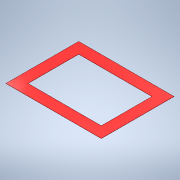
# Autodesk Inventor part: smt_keepout
Saved by Autodesk Inventor 2022 (Build 260153000, 153)
## iProperties
Created: 2022-02-26
Part Number: smt_keepout
Material: Generic
Document SubType Name: Modeling
Designer: Caleb
Density: 1 g/cm^3
Appearance: Light Red
Author: Caleb
Autodesk Inventor part; units mm, degrees
ref_plane "YZ Plane" through (0, 0, 0) normal (1, 0, 0) x (0, 1, 0)
ref_plane "XZ Plane" through (0, 0, 0) normal (0, 1, 0) x (-1, 0, 0)
ref_plane "XY Plane" through (0, 0, 0) normal (0, 0, 1) x (1, 0, 0)
sketch "Sketch1" plane through (0, 0, 0) normal (0, 1, 0) x (-1, 0, 0)
  line L0 (-28.25, -21.55) -> (28.25, -21.55)
  line L1 (28.25, -21.55) -> (28.25, 21.55)
  line L2 (28.25, 21.55) -> (-28.25, 21.55)
  line L3 (-28.25, 21.55) -> (-28.25, -21.55)
  line L4 (-28.25, -21.55) -> (28.25, 21.55) construction
  line L5 (28.25, -21.55) -> (-28.25, 21.55) construction
  point P0 (0, 0)
  dimension "d0" = 43.1
  dimension "d1" = 56.5
  constraints: 12 end point, 2 midpoint, 2 parallel, 1 horizontal, 1 perpendicular
  measures "d0" distance of L0.end L1.end
  measures "d1" distance of L1.end L2.end
extrude "Extrusion1" add sketch "Sketch1" along normal blind 0.1
sketch "Sketch2" plane through (0, 0.1, 0) normal (0, 1, 0) x (1, 0, 0)
  line L0 (21.75, 15.05) -> (-21.75, 15.05)
  line L1 (-21.75, 15.05) -> (-21.75, -15.05)
  line L2 (-21.75, -15.05) -> (21.75, -15.05)
  line L3 (21.75, -15.05) -> (21.75, 15.05)
  line L4 (21.75, 15.05) -> (-21.75, -15.05) construction
  line L5 (-21.75, 15.05) -> (21.75, -15.05) construction
  line L6 (-28.25, -21.55) -> (28.25, -21.55) projected
  line L7 (-28.25, 21.55) -> (-28.25, -21.55) projected
  point P0 (0, 0)
  dimension "d4" = 6.5
  dimension "d5" = 6.5
  constraints: 12 end point, 2 midpoint, 2 parallel, 1 horizontal, 1 perpendicular
  measures "d4" distance between parallel lines of L6 L2
  measures "d5" distance between parallel lines of L7 L1
extrude "Extrusion2" cut sketch "Sketch2" against normal through all
body "Solid1"
